slipring v2 (Autodesk Fusion 360 design; units mm, degrees)
Autodesk Fusion 360 part; units mm, degrees
sketch "Sketch1" plane through (0, 0, 0) normal (0, 0, 1) x (1, 0, 0)
  circle A0 centre (0, 0) radius 12
  circle A1 centre (0, 0) radius 9 construction
  line L0 (0, 0) -> (0, 12) construction
  circle A2 centre (0, 9) radius 1.6
  circle A3 centre (-7.7942, -4.5) radius 1.6
  circle A4 centre (7.7942, -4.5) radius 1.6
  circle A5 centre (0, 0) radius 2.5
  dimension "d1" = 24
  dimension "d2" = 18
  dimension "d3" = 3.2
  dimension "d5" = 360
  dimension "d6" = 5
  constraint coincident A0.centre A1.centre
  constraint concentric A0 A1
  constraint coincident A0 L0.end
  constraint vertical L0
  constraint coincident A1 A2.centre
  constraint coincident L0 A2.centre
  measures "d1" diameter of A0
  measures "d2" diameter of A1
  measures "d3" diameter of A2
  measures "d6" diameter of A5
extrude "Extrude1" add sketch "Sketch1" against normal blind 1.2 contours A0 | A5
extrude "Extrude2" add sketch "Sketch1" along normal blind 1.5 contours A5
sketch "Sketch3" plane through (0, 0, -1.2) normal (0, 0, -1) x (1, 0, 0)
  circle A0 centre (7.7942, 4.5) radius 1.6
  circle A1 centre (-7.7942, 4.5) radius 1.6
  circle A2 centre (0, -9) radius 1.6
  circle A3 centre (0, 0) radius 12
  circle A4 centre (0, 0) radius 6.25
  dimension "d14" = 12.5
  constraint concentric A3 A4
  measures "d14" diameter of A4
extrude "Extrude4" add sketch "Sketch3" along normal blind 13.8 contours A4
